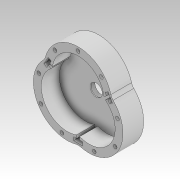
# Autodesk Inventor part: Housing
Saved by Autodesk Inventor 2020 (Build 240168000, 168)
## iProperties
Created: 2022-01-08
Part Number: Housing
Material: Generic
Document SubType Name: Modeling
Designer: DDeGo
Density: 1 g/cm^3
Appearance: Default
Author: DDeGo
Autodesk Inventor part; units mm, degrees
ref_plane "YZ Plane" through (0, 0, 0) normal (1, 0, 0) x (0, 1, 0)
ref_plane "XZ Plane" through (0, 0, 0) normal (0, 1, 0) x (-1, 0, 0)
ref_plane "XY Plane" through (0, 0, 0) normal (0, 0, 1) x (1, 0, 0)
derived "LP2_master.ipt"
sketch "ChamberWalls" plane through (0, 0, 0) normal (0, 0, 1) x (1, 0, 0)
  arc A0 (-8.6566, -4.9979) -> (14.9371, 8.624) centre (0, 7.2521) ccw construction
  arc A1 (0, -17.2479) -> (14.9371, 8.624) centre (6.2805, -3.626) ccw
  arc A2 (-14.9371, 8.624) -> (0, -17.2479) centre (-6.2805, -3.626) ccw
  line L0 (-6.2805, -3.626) -> (0, 0) construction
  line L1 (0, 0) -> (0, 7.2521) construction
  line L2 (0, 0) -> (6.2805, -3.626) construction
  arc A3 (0, 9.9958) -> (-14.9371, 8.624) centre (-6.2805, -3.626) ccw construction
  arc A4 (-14.9371, 8.624) -> (-8.6566, -4.9979) centre (0, 7.2521) ccw construction
  arc A5 (-8.6566, -4.9979) -> (0, -17.2479) centre (6.2805, -3.626) ccw construction
  arc A6 (0, -17.2479) -> (0, 9.9958) centre (-6.2805, -3.626) ccw construction
  arc A7 (14.9371, 8.624) -> (-14.9371, 8.624) centre (0, 7.2521) ccw
  arc A8 (14.9371, 8.624) -> (-8.6566, -4.9979) centre (6.2805, -3.626) ccw construction
  point P0 (19.2709, -11.126)
sketch "HousingWalls" plane through (0, 0, -1.5) normal (0, 0, 1) x (1, 0, 0)
  arc A0 (14.9371, 8.624) -> (-14.9371, 8.624) centre (0, 7.2521) ccw construction
  arc A1 (-14.9371, 8.624) -> (0, -17.2479) centre (-6.2805, -3.626) ccw construction
  arc A2 (0, -17.2479) -> (14.9371, 8.624) centre (6.2805, -3.626) ccw construction
  arc A3 (-20.1043, 10.1272) -> (-1.2817, -22.4744) centre (-6.2805, -3.626) ccw
  arc A4 (18.8226, 12.3472) -> (-18.8226, 12.3472) centre (0, 7.2521) ccw
  arc A5 (1.2817, -22.4744) -> (20.1043, 10.1272) centre (6.2805, -3.626) ccw
  arc A6 (-20.1043, 10.1272) -> (-18.8226, 12.3472) centre (-23.6489, 13.6537) ccw
  arc A7 (18.8226, 12.3472) -> (20.1043, 10.1272) centre (23.6489, 13.6537) ccw
  arc A8 (1.2817, -22.4744) -> (-1.2817, -22.4744) centre (0, -27.3074) ccw
  point P0 (0, 0)
sketch "ApexCut" plane through (0, 0, 0) normal (0, 0, 1) x (1, 0, 0)
  line L0 (0, 0) -> (-15.6733, 9.049) construction
  circle A0 centre (-15.6733, 9.049) radius 0.85 construction
  line L1 (-15.6733, 9.049) -> (-15.2483, 9.7851) construction
  line L2 (-15.2483, 9.7851) -> (-16.34, 10.4154)
  line L3 (-16.34, 10.4154) -> (-15.49, 11.8876)
  line L4 (-15.49, 11.8876) -> (-17.222, 12.8876)
  line L5 (-17.222, 12.8876) -> (-19.772, 8.4709)
  line L6 (-19.772, 8.4709) -> (-18.04, 7.4709)
  line L7 (-18.04, 7.4709) -> (-17.19, 8.9431)
  line L8 (-17.19, 8.9431) -> (-16.0983, 8.3128)
  line L9 (-17.19, 8.9431) -> (-16.34, 10.4154) construction
  line L10 (-16.0983, 8.3128) -> (-15.6733, 9.049) construction
  line L11 (-16.0983, 8.3128) -> (-15.3621, 7.8878)
  line L12 (-15.3621, 7.8878) -> (-14.5121, 9.3601)
  line L13 (-14.5121, 9.3601) -> (-15.2483, 9.7851)
  arc A1 (-14.9371, 8.624) -> (0, -17.2479) centre (-6.2805, -3.626) ccw construction
  point P0 (-15.6744, 8.0681)
ref_plane "Chamber_bot" through (0, 0, 0) normal (0, 0, 1) x (1, 0, 0)
ref_plane "Housing_bot" through (0, 0, -1.5) normal (0, 0, 1) x (1, 0, 0)
ref_plane "Rotor_bot" through (0, 0, -0.2) normal (0, 0, 1) x (1, 0, 0)
ref_plane "RotorFlat_bot" through (0, 0, 0.3) normal (0, 0, 1) x (1, 0, 0)
ref_plane "RotorTeeth_top" through (0, 0, 3) normal (0, 0, 1) x (1, 0, 0)
ref_plane "RotorTeeth_bot" through (0, 0, 0.5) normal (0, 0, 1) x (1, 0, 0)
ref_plane "RotorBearinggap" through (0, 0, 4) normal (0, 0, 1) x (1, 0, 0)
ref_plane "RotorBearing_bot" through (0, 0, 4.5) normal (0, 0, 1) x (1, 0, 0)
ref_plane "RotorBearing_top" through (0, 0, 8.5) normal (0, 0, 1) x (1, 0, 0)
ref_plane "RotorFlat_top" through (0, 0, 10.1) normal (0, 0, 1) x (1, 0, 0)
ref_plane "Chamber_top" through (0, 0, 10.4) normal (0, 0, 1) x (1, 0, 0)
ref_plane "HousingTeeth_top" through (0, 0, 2.5) normal (0, 0, 1) x (1, 0, 0)
sketch "HousingBoltPattern" plane through (0, 0, 10.4) normal (0, 0, 1) x (1, 0, 0)
  arc A0 (-20.1043, 10.1272) -> (-18.8226, 12.3472) centre (-23.6489, 13.6537) ccw construction
  arc A1 (18.8226, 12.3472) -> (-18.8226, 12.3472) centre (0, 7.2521) ccw construction
  arc A2 (-20.1043, 10.1272) -> (-1.2817, -22.4744) centre (-6.2805, -3.626) ccw construction
  arc A3 (18.8226, 12.3472) -> (20.1043, 10.1272) centre (23.6489, 13.6537) ccw construction
  arc A4 (1.2817, -22.4744) -> (20.1043, 10.1272) centre (6.2805, -3.626) ccw construction
  arc A5 (1.2817, -22.4744) -> (-1.2817, -22.4744) centre (0, -27.3074) ccw construction
  arc A6 (-14.9371, 8.624) -> (0, -17.2479) centre (-6.2805, -3.626) ccw construction
  arc A7 (14.9371, 8.624) -> (-14.9371, 8.624) centre (0, 7.2521) ccw construction
  arc A8 (0, -17.2479) -> (14.9371, 8.624) centre (6.2805, -3.626) ccw construction
  arc A9 (-17.1932, 9.9265) -> (0, -19.853) centre (-6.2805, -3.626) ccw construction
  arc A10 (0, -19.853) -> (17.1932, 9.9265) centre (6.2805, -3.626) ccw construction
  arc A11 (17.1932, 9.9265) -> (-17.1932, 9.9265) centre (0, 7.2521) ccw construction
  circle A12 centre (-22.6311, 2.3251) radius 1.05
  circle A13 centre (-21.3493, -12.326) radius 1.05
  circle A14 centre (-9.302, -20.7617) radius 1.05
  line L0 (-9.302, -20.7617) -> (-6.2805, -3.626) construction
  line L1 (-6.2805, -3.626) -> (-22.6311, 2.3251) construction
  line L2 (-6.2805, -3.626) -> (-21.3493, -12.326) construction
  line L3 (-6.2805, -3.626) -> (0, 0) construction
  circle A15 centre (9.302, -20.7617) radius 1.05
  circle A16 centre (21.3493, -12.326) radius 1.05
  circle A17 centre (22.6311, 2.3251) radius 1.05
  circle A18 centre (13.3292, 18.4366) radius 1.05
  circle A19 centre (0, 24.6521) radius 1.05
  circle A20 centre (-13.3292, 18.4366) radius 1.05
sketch "HousingBearing" plane through (0, 0, 0) normal (1, 0, 0) x (0, 1, 0)
  line L0 (0, 0) -> (0, -3.2)
  line L1 (0, -3.2) -> (4.025, -3.2)
  line L2 (4.025, -3.2) -> (4.525, -3.2)
  line L3 (4.525, -3.2) -> (6.551, -1.5)
  line L4 (6.551, -1.5) -> (6.551, 0) construction
  line L5 (6.551, 0) -> (3.525, 0) construction
  line L6 (4.025, -3.2) -> (4.025, -1.5)
  line L7 (4.025, -0.5) -> (3.525, -0.5)
  line L8 (3.525, -0.5) -> (3.525, 0)
  line L9 (-87.0508, -1.5) -> (84.6316, -1.5)
  line L10 (3.525, 0) -> (0, 0)
  line L11 (6.551, -1.5) -> (4.025, -1.5)
  line L12 (4.025, -1.5) -> (4.025, -0.5)
extrude "Extrusion1" add sketch "HousingWalls" along normal up to surface (1.5 mm away)
sketch "Sketch8" plane through (0, 7.2521, 0) normal (0, 0, 1) x (1, 0, 0)
  arc A0 (-14.9371, 1.3719) -> (0, -24.5) centre (-6.2805, -10.8781) ccw projected
  arc A1 (14.9371, 1.3719) -> (-14.9371, 1.3719) centre (0, 0) ccw projected
  arc A2 (0, -24.5) -> (14.9371, 1.3719) centre (6.2805, -10.8781) ccw projected
  arc A3 (-20.1043, 2.8751) -> (-1.2817, -29.7265) centre (-6.2805, -10.8781) ccw projected
  arc A4 (1.2817, -29.7265) -> (-1.2817, -29.7265) centre (0, -34.5595) ccw projected
  arc A5 (1.2817, -29.7265) -> (20.1043, 2.8751) centre (6.2805, -10.8781) ccw projected
  arc A6 (18.8226, 5.0952) -> (20.1043, 2.8751) centre (23.6489, 6.4016) ccw projected
  arc A7 (18.8226, 5.0952) -> (-18.8226, 5.0952) centre (0, 0) ccw projected
  arc A8 (-20.1043, 2.8751) -> (-18.8226, 5.0952) centre (-23.6489, 6.4016) ccw projected
  point P0 (0, -7.2521)
extrude "Extrusion2" add sketch "Sketch8" along normal up to surface (10.4 mm away)
extrude "Extrusion3" cut sketch "ApexCut" along normal through all
pattern_circular "Circular Pattern1" count 3 over 360 about axis through (0, 0, -1.5) along (0, 0, 1) of "Extrusion3"
extrude "Extrusion4" cut sketch "HousingBoltPattern" against normal through all
revolve "Revolution1" cut sketch "HousingBearing" angle 360 about axis through (0, 0, 0) along (0, 0, -1) contours L10 L8 L7 L12 L9 L0 | L9 L6 L1 L0
revolve "Revolution2" add sketch "HousingBearing" angle 360 about axis through (0, 0, 0) along (0, 0, -1) contours L9 L3 L2 L6
body "Solid1"
